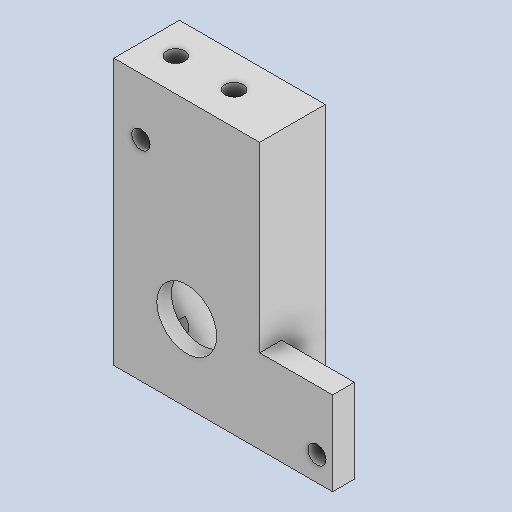
# Autodesk Inventor part: Soporte mecanismo 2
Saved by Autodesk Inventor 2023 (Build 270158000, 158)
## iProperties
Created: 2022-12-03
Part Number: Soporte mecanismo 2
Material: Genérico
Document SubType Name: Modeling
Designer: sergi
Density: 1 g/cm^3
Appearance: Valor por defecto
Author: sergi
Autodesk Inventor part; units mm, degrees
ref_plane "YZ Plane" through (0, 0, 0) normal (1, 0, 0) x (0, 1, 0)
ref_plane "XZ Plane" through (0, 0, 0) normal (0, 1, 0) x (-1, 0, 0)
ref_plane "Plano de trabajo1" through (-47.2143, 36.5, -75.5) normal (0, -1, 0) x (1, 0, 0)
sketch "Boceto1" plane through (0, 0, 0) normal (0, 1, 0) x (-1, 0, 0)
  line L0 (0, 0) -> (20, 0)
  line L1 (20, 0) -> (20, -9)
  line L2 (20, -9) -> (0, -9)
  line L3 (0, -9) -> (0, 0)
  line L4 (0, 0) -> (-10, 0)
  line L5 (-10, 0) -> (-10, -3)
  line L6 (-10, -3) -> (0, -3)
  line L7 (0, -3) -> (0, 0)
  dimension "d0" = 20
  dimension "d1" = 9
  dimension "d25" = 10
  dimension "d26" = 3
  constraints: 16 end point, 4 parallel, 2 horizontal, 2 perpendicular
  measures "d0" distance of L1.end L2.end
  measures "d1" distance of L0.end L1.end
  measures "d25" distance of L6.end L5.end
  measures "d26" distance of L5.end L4.end
extrude "Extrusión1" add sketch "Boceto1" along normal up to surface (36.5 mm away)
sketch "Boceto2" plane through (0, 0, -9) normal (0, 0, -1) x (-1, 0, 0)
  circle A0 centre (10, 10.5) radius 4.5 projected
  point P0 (0, 0)
hole "Agujero1" at (-10, 10.5, -9) direction (0, 0, 1) diameter 16.2 depth 7
sketch "Boceto3" plane through (0, 0, -9) normal (0, 0, -1) x (-1, 0, 0)
  circle A0 centre (10, 10.5) radius 8.1 projected
  point P0 (0, 0)
  constraints: 1 coincident
hole "Agujero2" at (-10, 10.5, -9) direction (0, 0, 1) diameter 8.2 end through all
sketch "Boceto4" plane through (0, 0, 0) normal (0, -1, 0) x (1, 0, 0)
  circle A0 centre (-4, -4.5) radius 1.25 projected
  circle A1 centre (-16, -4.5) radius 1.25 projected
  point P0 (0, 0)
hole "Agujero3" at (-16, 0, -4.5) at (-4, 0, -4.5) direction (0, 1, 0) diameter 2.5 depth 5
sketch "Boceto6" plane through (-20, 36.5, 0) normal (0, 1, 0) x (1, 0, 0)
  line L0 (30, 0) -> (30, 3) projected
  line L1 (30, 3) -> (20, 3)
  line L2 (20, 3) -> (20, 0)
  line L3 (20, 0) -> (30, 0)
  line L4 (30, 0) -> (30, 3)
  constraints: 8 end point, 2 parallel, 1 horizontal, 1 perpendicular
extrude "Extrusión2" cut sketch "Boceto6" against normal blind 25
sketch "Boceto7" plane through (-20, 0, 0) normal (0, 0, 1) x (1, 0, 0)
  circle A0 centre (3.7217, 28.6888) radius 2.1 projected
  circle A1 centre (27.863, 3.3471) radius 2.1 projected
  circle A2 centre (3.7217, 28.6888) radius 1.25
  circle A3 centre (27.863, 3.3471) radius 1.25
  point P0 (20, 0)
  dimension "d31" = 2.5
  dimension "d32" = 2.5
  constraints: 2 centre point, 2 coincident
  measures "d31" diameter of A2
  measures "d32" diameter of A3
extrude "Extrusión3" cut sketch "Boceto7" against normal through all contours A2 | A3
sketch "Boceto8" plane through (-20, 36.5, -9) normal (0, 1, 0) x (1, 0, 0)
  line L0 (0, 0) -> (0, -9) projected
  line L1 (0, -4.5) -> (4, -4.5)
  line L2 (4, -4.5) -> (12, -4.5)
  circle A0 centre (4, -4.5) radius 1.25
  circle A1 centre (12, -4.5) radius 1.25
  point P0 (20, -9)
  dimension "d33" = 4
  dimension "d34" = 8
  dimension "d35" = 2.5
  constraints: 4 end point, 2 centre point, 2 coincident, 1 horizontal, 1 midpoint, 1 point on line
  measures "d33" distance of L1.start L1.end
  measures "d34" distance of L1.end L2.end
  measures "d35" diameter of A0
extrude "Extrusión4" cut sketch "Boceto8" against normal blind 10
